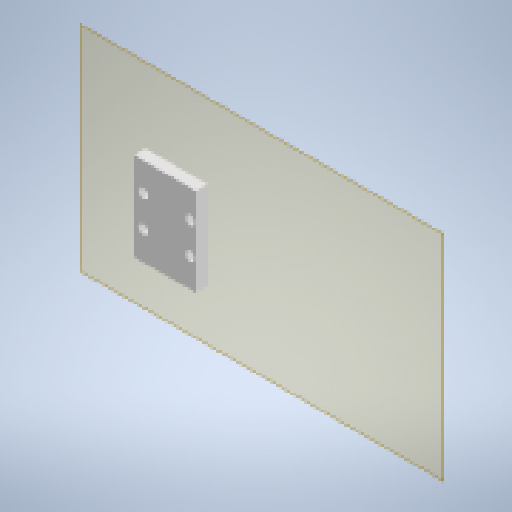
# Autodesk Inventor part: проставк
Saved by Autodesk Inventor 2024.2 (Build 282272000, 272)
## iProperties
Created: 2025-12-30
Part Number: проставк
Material: Типовые
Document SubType Name: Modeling
Designer: katya_notebook
Density: 1 g/cm^3
Appearance: По умолчанию
Author: katya_notebook
Autodesk Inventor part; units mm, degrees
ref_plane "YZ Plane" through (0, 0, 0) normal (1, 0, 0) x (0, 1, 0)
ref_plane "XZ Plane" through (0, 0, 0) normal (0, 1, 0) x (-1, 0, 0)
ref_plane "XY Plane" through (0, 0, 0) normal (0, 0, 1) x (1, 0, 0)
ref_plane "РабПлоскость1" through (51.8181, -3.2568, 14.8616) normal (0, 0, 1) x (1, 0, 0)
sketch "Эскиз1" plane through (51.8181, -3.2568, 14.8616) normal (0, 0, 1) x (1, 0, 0)
  line L0 (-26.6721, 3.7827) -> (-26.6721, -9.7173)
  line L1 (-30.7721, 8.2755) -> (-13.9721, 8.2755)
  line L2 (-13.9721, 8.2755) -> (-13.9721, -14.4178)
  line L3 (-13.9721, -14.4178) -> (-30.7721, -14.4178)
  line L4 (-30.7721, -14.4178) -> (-30.7721, 8.2755)
  point P0 (-51.8181, 3.2568)
  constraints: 10 end point, 2 parallel, 1 horizontal, 1 perpendicular, 1 vertical, 2 other
extrude "Выдавливание1" add sketch "Эскиз1" along normal blind 3
sketch "Эскиз2" plane through (51.8181, -3.2568, 14.8616) normal (0, 0, -1) x (-1, 0, 0)
  circle A0 centre (27.4758, 1.0327) radius 1.2
  circle A1 centre (15.4758, 1.0327) radius 1.2
  circle A2 centre (15.4758, -6.9673) radius 1.2
  circle A3 centre (27.4758, -6.9673) radius 1.2
  point P0 (51.8181, 3.2568)
  constraints: 4 centre point
extrude "Выдавливание2" cut sketch "Эскиз2" against normal blind 10
sketch "Эскиз3" plane through (51.8181, -3.2568, 14.8616) normal (0, 0, -1) x (-1, 0, 0)
  line L0 (30.7721, -14.4178) -> (13.9721, -14.4178) projected
  line L1 (13.9721, -14.4178) -> (28.9801, -14.4178)
  line L2 (28.9801, -14.4178) -> (28.9801, 8.2755)
  line L3 (28.9801, 8.2755) -> (13.9721, 8.2755)
  line L4 (13.9721, 8.2755) -> (13.9721, -14.4178)
  line L5 (13.9721, 8.2755) -> (30.7721, 8.2755) projected
  line L6 (30.7721, -14.4178) -> (28.9801, -14.4178)
  line L7 (28.9801, -14.4178) -> (28.9801, 8.2755)
  line L8 (28.9801, 8.2755) -> (30.7721, 8.2755)
  line L9 (30.7721, 8.2755) -> (30.7721, -14.4178)
  point P0 (51.8181, 3.2568)
  point P1 (30.7721, 8.2755)
  point P2 (28.9801, 8.2755)
  dimension "d4" = 15.008
  constraints: 16 end point, 4 parallel, 2 horizontal, 2 perpendicular, 1 point on line
  measures "d4" distance of L3.end L2.end
extrude "Выдавливание3" cut sketch "Эскиз3" against normal blind 10 contours L0 L2 L5 L9
